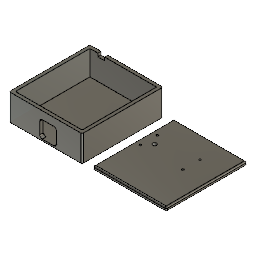
Bluetooth Box v1 (Autodesk Fusion 360 design; units mm, degrees)
Autodesk Fusion 360 part; units mm, degrees
box "BoxPrimitive1" add length 125 width 113 height 40 placed x (0, 1, 0) y (-1, 0, 0) z (0, 0, 1) at (102.5, 42.5, 0) makes body 1
shell "Shell1" thickness 5 removed faces 1 at (27.1667, 84.1667, 40) on bodies 1
fillet "Fillet1" radius 2 4 edges at (102.5, 167.5, 20) (-10.5, 167.5, 20) (-10.5, 42.5, 20) (102.5, 42.5, 20) on bodies 1
fillet "Fillet2" radius 2 1 faces at (64.8333, 125.1667, 0) on bodies 1
sketch "Sketch2" plane through (0, 42.5, 0) normal (0, -1, 0) x (1, 0, 0)
  line L0 (-8.5, 2) -> (100.5, 2)
  line L1 (100.5, 2) -> (100.5, 40)
  line L2 (100.5, 40) -> (-8.5, 40)
  line L3 (-8.5, 40) -> (-8.5, 2)
  line L4 (37, 25) -> (37, 15)
  line L5 (41, 2) -> (59, 2)
  line L6 (63, 6) -> (63, 24)
  line L7 (59, 28) -> (41, 28)
  line L8 (37, 24) -> (37, 6)
  arc A0 (41, 28) -> (37, 24) centre (41, 24) ccw
  arc A1 (37, 6) -> (41, 2) centre (41, 6) ccw
  arc A2 (59, 2) -> (63, 6) centre (59, 6) ccw
  arc A3 (63, 24) -> (59, 28) centre (59, 24) ccw
  point P0 (37, 2)
  point P1 (63, 2)
  point P2 (37, 28)
  dimension "d9" = 26
  dimension "d10" = 26
  dimension "d11" = 4
  dimension "d12" = 4
  dimension "d13" = 4
  dimension "d14" = 4
  constraint vertical L4
  constraint horizontal L5
  constraint vertical L6
  constraint vertical L8
  constraint coincident L0 P0
  constraint coincident P2 L7
  constraint coincident P2 L8
  constraint tangent L7 A0
  constraint tangent L8 A0
  constraint coincident P0 L5
  constraint coincident P0 L8
  constraint tangent L5 A1
  constraint tangent L8 A1
  constraint coincident P1 L5
  constraint coincident P1 L6
  constraint tangent L5 A2
  constraint tangent L6 A2
  constraint tangent L6 A3
  constraint tangent L7 A3
  measures "d9" distance of P0 P1
  measures "d10" distance of P0 P2
  measures "d11" radius of A0
  measures "d12" radius of A1
  measures "d13" radius of A2
  measures "d14" radius of A3
extrude "Extrude1" cut sketch "Sketch2" against normal blind 6 contours L0 L4 L5 L6 L7 L8 A0 A1 A2 A3 bodies 1
fillet "Fillet4" radius 2 1 edges at (-5.5, 47.5, 22.5) on bodies 1
fillet "Fillet5" radius 2 1 edges at (97.5, 47.5, 22.5) on bodies 1
sketch "Sketch3" plane through (0, 0, 40) normal (0, 0, 1) x (-1, 0, 0)
  arc A0 (-100.5, -42.5) -> (-102.5, -44.5) centre (-100.5, -44.5) ccw
  line L0 (-102.5, -44.5) -> (-102.5, -165.5)
  arc A1 (-102.5, -165.5) -> (-100.5, -167.5) centre (-100.5, -165.5) ccw
  line L1 (-100.5, -167.5) -> (8.5, -167.5)
  arc A2 (8.5, -167.5) -> (10.5, -165.5) centre (8.5, -165.5) ccw
  line L2 (10.5, -165.5) -> (10.5, -44.5)
  arc A3 (10.5, -44.5) -> (8.5, -42.5) centre (8.5, -44.5) ccw
  line L3 (8.5, -42.5) -> (-100.5, -42.5)
  line L4 (-97.5, -162.5) -> (-97.5, -49.5)
  arc A4 (-95.5, -47.5) -> (-97.5, -49.5) centre (-95.5, -49.5) ccw
  line L5 (-95.5, -47.5) -> (3.5, -47.5)
  arc A5 (5.5, -49.5) -> (3.5, -47.5) centre (3.5, -49.5) ccw
  line L6 (5.5, -49.5) -> (5.5, -162.5)
  line L7 (5.5, -162.5) -> (-97.5, -162.5)
  line L8 (-6.8903, -167.5) -> (-16.8903, -167.5)
  line L9 (-16.8903, -167.5) -> (-16.8903, -165)
  line L10 (-16.8903, -165) -> (-6.8903, -165)
  line L11 (-6.8903, -165) -> (-6.8903, -167.5)
  dimension "d20" = 10
  dimension "d21" = 2.5
  constraint horizontal L8
  constraint vertical L9
  constraint horizontal L10
  constraint vertical L11
  constraint coincident L1 L8.start
  measures "d20" distance of L8.start L8.end
  measures "d21" distance of L8.start L10.end
sketch "Sketch4" plane through (0, 0, 40) normal (0, 0, 1) x (-1, 0, 0)
sketch "Sketch5" plane through (0, 0, 40) normal (0, 0, 1) x (-1, 0, 0)
extrude "Extrude2" cut sketch "Sketch3" against normal blind 5 contours L1 L8 L9 L10 L11 bodies 1
box "BoxPrimitive2" add length 113 width 125 height 5 placed x (0, 1, 0) y (-1, 0, 0) z (0, 0, 1) at (240.4583, 61.2182, 0) separate body makes body 2
move_body "Move1" bodies 2 to x (0, -1, 0) y (1, 0, 0) z (0, 0, 1) at (54.2401, 286.6765, 0)
fillet "Fillet6" radius 2 4 edges at (228.4583, 46.2182, 2.5) (228.4583, 171.2182, 2.5) (115.4583, 171.2182, 2.5) (115.4583, 46.2182, 2.5) on bodies 2
sketch "Sketch7" plane through (-10.5, 0, 0) normal (-1, 0, 0) x (0, -1, 0)
  line L0 (-165.5, 2) -> (-44.5, 2)
  line L1 (-44.5, 2) -> (-44.5, 40)
  line L2 (-44.5, 40) -> (-165.5, 40)
  line L3 (-165.5, 40) -> (-165.5, 2)
sketch "Sketch8" plane through (0, 0, 5) normal (0, 0, 1) x (-1, 0, 0)
  arc A0 (-115.4583, -48.2182) -> (-117.4583, -46.2182) centre (-117.4583, -48.2182) ccw
  line L0 (-117.4583, -46.2182) -> (-226.4583, -46.2182)
  arc A1 (-226.4583, -46.2182) -> (-228.4583, -48.2182) centre (-226.4583, -48.2182) ccw
  line L1 (-228.4583, -48.2182) -> (-228.4583, -169.2182)
  arc A2 (-228.4583, -169.2182) -> (-226.4583, -171.2182) centre (-226.4583, -169.2182) ccw
  line L2 (-226.4583, -171.2182) -> (-117.4583, -171.2182)
  arc A3 (-117.4583, -171.2182) -> (-115.4583, -169.2182) centre (-117.4583, -169.2182) ccw
  line L3 (-115.4583, -169.2182) -> (-115.4583, -48.2182)
  circle A4 centre (-125, -110) radius 1.5
  circle A5 centre (-125.0173, -136.2474) radius 1.5
  circle A6 centre (-190.7477, -136.2474) radius 1.5
  circle A7 centre (-190.7477, -109.9581) radius 1.5
  circle A8 centre (-135, -122) radius 3
  dimension "d30" = 3
  dimension "d31" = 3
  dimension "d32" = 3
  dimension "d33" = 3
  dimension "d34" = 6
  measures "d30" diameter of A4
  measures "d31" diameter of A5
  measures "d32" diameter of A6
  measures "d33" diameter of A7
  measures "d34" diameter of A8
extrude "Extrude3" cut sketch "Sketch8" against normal blind 5 contours A4 | A5 | A6 | A7 | A8 bodies 2
move_face "OffsetFaces1" offset 2.5 1 faces at (27.8333, 84.8333, 0) on bodies 1
move_body "Move2" bodies 1 to x (1, 0, 0) y (0, 1, 0) z (0, 0, 1) at (0, 0, 2.5)
move_face "OffsetFaces2" offset -3 1 faces at (13.557, 165, 40.8333) on bodies 1
extrude "Extrude4" cut 1 faces at (43.0423, 124.5, 7.5) along direction (0, 0, -1) blind 3 on bodies 1 bodies 1
fillet "Fillet7" radius 2 8 edges at (116.0441, 170.6324, 5) (115.4583, 108.7182, 5) (116.0441, 46.804, 5) (171.9583, 46.2182, 5) (227.8725, 46.804, 5) (228.4583, 108.7182, 5) (227.8725, 170.6324, 5) (171.9583, 171.2182, 5) on bodies 2
